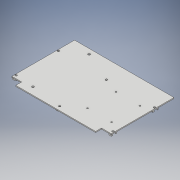
# Autodesk Inventor part: PiAndBusBarPlate
Saved by Autodesk Inventor 2018.3 (Build 223284000, 284)
## iProperties
Created: 2019-03-27
Part Number: PiAndBusBarPlate
Material: Generic
Document SubType Name: Modeling
Designer: matth
Density: 1 g/cm^3
Appearance: Default
Author: matth
Autodesk Inventor part; units mm, degrees
ref_plane "YZ Plane" through (0, 0, 0) normal (1, 0, 0) x (0, 1, 0)
ref_plane "XZ Plane" through (0, 0, 0) normal (0, 1, 0) x (-1, 0, 0)
ref_plane "XY Plane" through (0, 0, 0) normal (0, 0, 1) x (1, 0, 0)
sketch "Sketch1" plane through (0, 0, 0) normal (0, 0, 1) x (1, 0, 0)
  line L0 (-58.4998, -9.3705) -> (144.5002, -9.3705)
  line L1 (144.5002, -9.3705) -> (144.5002, -119.3705)
  line L2 (144.5002, -119.3705) -> (-58.4998, -119.3705)
  line L3 (-58.4998, -119.3705) -> (-58.4998, -9.3705)
  line L4 (-58.4998, -9.3705) -> (-38.4998, -9.3705)
  line L5 (-38.4998, -9.3705) -> (-38.4998, -21.3705)
  line L6 (-38.4998, -21.3705) -> (-58.4998, -21.3705)
  line L7 (-58.4998, -21.3705) -> (-58.4998, -9.3705)
  line L8 (144.5002, -9.3705) -> (124.5002, -9.3705)
  line L9 (124.5002, -9.3705) -> (124.5002, -21.3705)
  line L10 (124.5002, -21.3705) -> (144.5002, -21.3705)
  line L11 (144.5002, -21.3705) -> (144.5002, -9.3705)
  circle A0 centre (-56.009, -27.3705) radius 2
  circle A1 centre (142.0094, -27.3705) radius 2
  circle A2 centre (43.0002, -17.3705) radius 2
  circle A3 centre (-56.009, -111.8705) radius 2
  circle A4 centre (42.0002, -111.8705) radius 2
  circle A5 centre (142.0094, -113.8705) radius 2
  point P0 (0, 0)
  dimension "d0" = 203
  dimension "d1" = 110
  dimension "d2" = 20
  dimension "d3" = 12
  dimension "d4" = 20
  dimension "d5" = 12
  dimension "d6" = 4
  dimension "d7" = 4
  dimension "d8" = 198.0184
  dimension "d9" = 2.4908
  dimension "d10" = 18
  dimension "d11" = 4
  dimension "d12" = 10
  dimension "d13" = 99.0092
  dimension "d14" = 4
  dimension "d15" = 84.5
  dimension "d16" = 4
  dimension "d17" = 4
  dimension "d18" = 0
  constraints: 24 end point, 6 centre point, 6 parallel, 3 horizontal, 3 perpendicular
  measures "d0" distance of L1.end L2.end
  measures "d1" distance of L0.end L1.end
  measures "d2" distance of L5.end L6.end
  measures "d3" distance of L4.end L5.end
  measures "d4" distance of L10.end L9.end
  measures "d5" distance of L9.end L8.end
  measures "d6" diameter of A0
  measures "d7" diameter of A1
  measures "d8" distance of A1.centre A0.centre
  measures "d9" distance from line of L3 A0.centre
  measures "d10" distance from line of L0 A0.centre
  measures "d11" diameter of A2
  measures "d12" vertical distance of A0.centre A2.centre
  measures "d13" horizontal distance of A0.centre A2.centre
  measures "d14" diameter of A3
  measures "d15" distance of A0.centre A3.centre
  measures "d16" diameter of A4
  measures "d17" diameter of A5
  measures "d18" horizontal distance of A1.centre A5.centre
extrude "Extrusion1" add sketch "Sketch1" along normal blind 2 contours L0 L9 L10 L1 L2 L3 L6 L5
sketch "Sketch3" plane through (0, 0, 0) normal (0, 0, -1) x (-1, 0, 0)
  circle A0 centre (56.009, -111.8705) radius 2 projected
  circle A1 centre (-42.0002, -111.8705) radius 2 projected
  circle A2 centre (-142.0094, -113.8705) radius 2 projected
  circle A3 centre (-142.0094, -27.3705) radius 2 projected
  circle A4 centre (-43.0002, -17.3705) radius 2 projected
  circle A5 centre (56.009, -27.3705) radius 2 projected
  circle A6 centre (56.009, -111.8705) radius 6
  circle A7 centre (-42.0002, -111.8705) radius 6
  circle A8 centre (-142.0094, -113.8705) radius 2 projected
  circle A9 centre (-142.0094, -113.8705) radius 6
  circle A10 centre (-43.0002, -17.3705) radius 6
  circle A11 centre (-142.0094, -27.3705) radius 6
  circle A12 centre (56.009, -27.3705) radius 6
  circle A13 centre (56.009, -111.8705) radius 4
  circle A14 centre (-42.0002, -111.8705) radius 4
  circle A15 centre (56.009, -27.3705) radius 4
  circle A16 centre (-43.0002, -17.3705) radius 4
  circle A17 centre (-142.0094, -27.3705) radius 4
  circle A18 centre (-142.0094, -113.8705) radius 4
  point P0 (0, 0)
  dimension "d45" = 12
  dimension "d46" = 12
  dimension "d47" = 12
  dimension "d48" = 12
  dimension "d49" = 12
  dimension "d50" = 12
  dimension "d51" = 8
  dimension "d52" = 8
  dimension "d53" = 8
  dimension "d54" = 8
  dimension "d55" = 8
  dimension "d56" = 8
  constraints: 12 centre point, 12 coincident
  measures "d45" diameter of A6
  measures "d46" diameter of A7
  measures "d47" diameter of A9
  measures "d48" diameter of A10
  measures "d49" diameter of A11
  measures "d50" diameter of A12
  measures "d51" diameter of A13
  measures "d52" diameter of A14
  measures "d53" diameter of A15
  measures "d54" diameter of A16
  measures "d55" diameter of A17
  measures "d56" diameter of A18
extrude "Extrusion3" add sketch "Sketch3" along normal blind 3 contours A6 | A7 | A9 | A10 | A11 | A12
sketch "Sketch4" plane through (0, 0, 2) normal (0, 0, 1) x (1, 0, 0)
  line L0 (124.5002, -9.3705) -> (-38.4998, -9.3705) projected
  line L1 (-38.4998, -9.3705) -> (-38.4998, -21.3705) projected
  line L2 (-38.4998, -21.3705) -> (-58.4998, -21.3705) projected
  line L3 (-58.4998, -21.3705) -> (-58.4998, -119.3705) projected
  line L4 (-58.4998, -119.3705) -> (144.5002, -119.3705) projected
  line L5 (144.5002, -119.3705) -> (144.5002, -21.3705) projected
  line L6 (144.5002, -21.3705) -> (124.5002, -21.3705) projected
  line L7 (124.5002, -21.3705) -> (124.5002, -9.3705) projected
  line L8 (-77.131, 13.4165) -> (211.8208, 13.4165)
  line L9 (211.8208, 13.4165) -> (211.8208, -174.2275)
  line L10 (211.8208, -174.2275) -> (-77.131, -174.2275)
  line L11 (-77.131, -174.2275) -> (-77.131, 13.4165)
  point P0 (0, 0)
  constraints: 8 end point, 2 parallel, 1 horizontal, 1 perpendicular
extrude "Extrusion4" cut sketch "Sketch4" against normal through all
sketch "Sketch6" plane through (0, 0, 2) normal (0, 0, 1) x (1, 0, 0)
  circle A0 centre (-38.4998, -99.9669) radius 1.5
  circle A1 centre (-38.4998, -41.9669) radius 1.5
  line L0 (-58.4998, -21.3705) -> (-58.4998, -119.3705) projected
  circle A2 centre (10.5002, -99.9669) radius 1.5
  circle A3 centre (10.5002, -41.9669) radius 1.5
  point P0 (0, 0)
  dimension "d73" = 3
  dimension "d74" = 3
  dimension "d75" = 20
  dimension "d76" = 20
  dimension "d77" = 58
  dimension "d78" = 3
  dimension "d79" = 49
  dimension "d80" = 3
  constraints: 4 centre point
  measures "d73" diameter of A0
  measures "d74" diameter of A1
  measures "d75" distance from line of L0 A1.centre
  measures "d76" distance from line of L0 A0.centre
  measures "d77" distance of A1.centre A0.centre
  measures "d78" diameter of A2
  measures "d79" distance of A0.centre A2.centre
  measures "d80" diameter of A3
extrude "Extrusion6" cut sketch "Sketch6" against normal blind 10
sketch "Sketch8" plane through (0, 0, 2) normal (0, 0, 1) x (1, 0, 0)
  line L0 (-58.4998, -119.3705) -> (144.5002, -119.3705) projected
  line L1 (144.5002, -119.3705) -> (-58.4998, -119.3705)
  line L2 (-58.4998, -119.3705) -> (-58.4998, -149.3705)
  line L3 (-58.4998, -149.3705) -> (144.5002, -149.3705)
  line L4 (144.5002, -149.3705) -> (144.5002, -119.3705)
  point P0 (0, 0)
  dimension "d86" = 30
  constraints: 8 end point, 2 parallel, 1 horizontal, 1 perpendicular
  measures "d86" distance of L2.end L1.end
extrude "Extrusion7" add sketch "Sketch8" against normal blind 2
sketch "Sketch9" plane through (0, 0, 2) normal (0, 0, 1) x (1, 0, 0)
  circle A0 centre (104.5002, -24.3705) radius 2.25
  circle A1 centre (104.5002, -139.0705) radius 2.25
  line L0 (124.5002, -9.3705) -> (-38.4998, -9.3705) projected
  line L1 (144.5002, -149.3705) -> (144.5002, -21.3705) projected
  point P0 (0, 0)
  dimension "d89" = 4.5
  dimension "d90" = 4.5
  dimension "d91" = 15
  dimension "d92" = 114.7
  dimension "d93" = 40
  dimension "d94" = 40
  constraints: 2 centre point
  measures "d89" diameter of A0
  measures "d90" diameter of A1
  measures "d91" distance from line of L0 A0.centre
  measures "d92" distance of A0.centre A1.centre
  measures "d93" distance from line of L1 A0.centre
  measures "d94" distance from line of L1 A1.centre
extrude "Extrusion8" cut sketch "Sketch9" against normal blind 2
equation "\"d13\" = 0.5 * d8"
body "Solid1"
